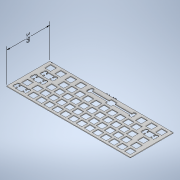
# Autodesk Inventor part: plate
Saved by Autodesk Inventor 2022 (Build 260153000, 153)
## iProperties
Created: 2022-03-03
Part Number: plate
Material: Generic
Document SubType Name: Modeling
Designer: Nathan Griffith
Density: 1 g/cm^3
Appearance: Machined - Aluminum
Author: Nathan Griffith
Autodesk Inventor part; units mm, degrees
ref_plane "YZ Plane" through (0, 0, 0) normal (1, 0, 0) x (0, 1, 0)
ref_plane "XZ Plane" through (0, 0, 0) normal (0, 1, 0) x (-1, 0, 0)
ref_plane "XY Plane" through (0, 0, 0) normal (0, 0, 1) x (1, 0, 0)
sketch "Sketch1" plane through (0, 0, 0) normal (0, 1, 0) x (-1, 0, 0)
  line L0 (0.0951, 101.505) -> (291.845, 101.505)
  line L1 (291.845, 101.505) -> (291.845, 0.2549)
  line L2 (291.845, 0.2549) -> (0.0951, 0.2549)
  line L3 (0.0951, 0.2549) -> (0.0951, 101.505)
  line L4 (127.062, 19.7804) -> (127.062, 15.0799)
  line L5 (127.062, 15.0799) -> (87.4377, 15.0799)
  line L6 (87.4377, 15.0799) -> (87.4377, 18.31)
  line L7 (87.4377, 18.31) -> (80.687, 18.31)
  line L8 (80.687, 18.31) -> (80.687, 15.0799)
  line L9 (80.687, 15.0799) -> (79.8629, 15.0799)
  line L10 (79.8629, 15.0799) -> (79.8629, 12.2811)
  line L11 (79.8629, 12.2811) -> (80.687, 12.2811)
  line L12 (80.687, 12.2811) -> (80.687, 6.011)
  line L13 (80.687, 6.011) -> (82.4121, 6.011)
  line L14 (82.4121, 6.011) -> (82.4121, 4.8107)
  line L15 (82.4121, 4.8107) -> (85.7127, 4.8107)
  line L16 (85.7127, 4.8107) -> (85.7127, 6.011)
  line L17 (85.7127, 6.011) -> (87.4377, 6.011)
  line L18 (87.4377, 6.011) -> (87.4377, 10.4813)
  line L19 (87.4377, 10.4813) -> (127.062, 10.4813)
  line L20 (127.062, 10.4813) -> (127.062, 5.7809)
  line L21 (127.062, 5.7809) -> (141.063, 5.7809)
  line L22 (141.063, 5.7809) -> (141.063, 10.4813)
  line L23 (141.063, 10.4813) -> (180.687, 10.4813)
  line L24 (180.687, 10.4813) -> (180.687, 6.011)
  line L25 (180.687, 6.011) -> (182.412, 6.011)
  line L26 (182.412, 6.011) -> (182.412, 4.8107)
  line L27 (182.412, 4.8107) -> (185.713, 4.8107)
  line L28 (185.713, 4.8107) -> (185.713, 6.011)
  line L29 (185.713, 6.011) -> (187.438, 6.011)
  line L30 (187.438, 6.011) -> (187.438, 12.2811)
  line L31 (187.438, 12.2811) -> (188.262, 12.2811)
  line L32 (188.262, 12.2811) -> (188.262, 15.0799)
  line L33 (188.262, 15.0799) -> (187.438, 15.0799)
  line L34 (187.438, 15.0799) -> (187.438, 18.31)
  line L35 (187.438, 18.31) -> (180.687, 18.31)
  line L36 (180.687, 18.31) -> (180.687, 15.0799)
  line L37 (180.687, 15.0799) -> (141.063, 15.0799)
  line L38 (141.063, 15.0799) -> (141.063, 19.7804)
  line L39 (141.063, 19.7804) -> (127.062, 19.7804)
  line L40 (269.937, 19.7804) -> (283.938, 19.7804)
  line L41 (283.938, 19.7804) -> (283.938, 5.7809)
  line L42 (283.938, 5.7809) -> (269.937, 5.7809)
  line L43 (269.937, 5.7809) -> (269.937, 19.7804)
  line L44 (246.126, 19.7804) -> (260.125, 19.7804)
  line L45 (260.125, 19.7804) -> (260.125, 5.7809)
  line L46 (260.125, 5.7809) -> (246.126, 5.7809)
  line L47 (246.126, 5.7809) -> (246.126, 19.7804)
  line L48 (222.312, 19.7804) -> (236.313, 19.7804)
  line L49 (236.313, 19.7804) -> (236.313, 5.7809)
  line L50 (236.313, 5.7809) -> (222.312, 5.7809)
  line L51 (222.312, 5.7809) -> (222.312, 19.7804)
  line L52 (198.501, 19.7804) -> (212.5, 19.7804)
  line L53 (212.5, 19.7804) -> (212.5, 5.7809)
  line L54 (212.5, 5.7809) -> (198.501, 5.7809)
  line L55 (198.501, 5.7809) -> (198.501, 19.7804)
  line L56 (55.626, 19.7804) -> (69.6253, 19.7804)
  line L57 (69.6253, 19.7804) -> (69.6253, 5.7809)
  line L58 (69.6253, 5.7809) -> (55.626, 5.7809)
  line L59 (55.626, 5.7809) -> (55.626, 19.7804)
  line L60 (31.812, 19.7804) -> (45.8128, 19.7804)
  line L61 (45.8128, 19.7804) -> (45.8128, 5.7809)
  line L62 (45.8128, 5.7809) -> (31.812, 5.7809)
  line L63 (31.812, 5.7809) -> (31.812, 19.7804)
  line L64 (8.0009, 19.7804) -> (22.0004, 19.7804)
  line L65 (22.0004, 19.7804) -> (22.0004, 5.7809)
  line L66 (22.0004, 5.7809) -> (8.0009, 5.7809)
  line L67 (8.0009, 5.7809) -> (8.0009, 19.7804)
  line L68 (255.65, 38.8303) -> (255.65, 34.1299)
  line L69 (255.65, 34.1299) -> (254.125, 34.1299)
  line L70 (254.125, 34.1299) -> (254.125, 37.3599)
  line L71 (254.125, 37.3599) -> (247.376, 37.3599)
  line L72 (247.376, 37.3599) -> (247.376, 34.1299)
  line L73 (247.376, 34.1299) -> (246.55, 34.1299)
  line L74 (246.55, 34.1299) -> (246.55, 31.3311)
  line L75 (246.55, 31.3311) -> (247.376, 31.3311)
  line L76 (247.376, 31.3311) -> (247.376, 25.061)
  line L77 (247.376, 25.061) -> (249.101, 25.061)
  line L78 (249.101, 25.061) -> (249.101, 23.8607)
  line L79 (249.101, 23.8607) -> (252.4, 23.8607)
  line L80 (252.4, 23.8607) -> (252.4, 25.061)
  line L81 (252.4, 25.061) -> (254.125, 25.061)
  line L82 (254.125, 25.061) -> (254.125, 29.53)
  line L83 (254.125, 29.53) -> (255.65, 29.53)
  line L84 (255.65, 29.53) -> (255.65, 24.8309)
  line L85 (255.65, 24.8309) -> (269.65, 24.8309)
  line L86 (269.65, 24.8309) -> (269.65, 29.53)
  line L87 (269.65, 29.53) -> (271.176, 29.53)
  line L88 (271.176, 29.53) -> (271.176, 25.061)
  line L89 (271.176, 25.061) -> (272.901, 25.061)
  line L90 (272.901, 25.061) -> (272.901, 23.8607)
  line L91 (272.901, 23.8607) -> (276.2, 23.8607)
  line L92 (276.2, 23.8607) -> (276.2, 25.061)
  line L93 (276.2, 25.061) -> (277.925, 25.061)
  line L94 (277.925, 25.061) -> (277.925, 31.3311)
  line L95 (277.925, 31.3311) -> (278.751, 31.3311)
  line L96 (278.751, 31.3311) -> (278.751, 34.1299)
  line L97 (278.751, 34.1299) -> (277.925, 34.1299)
  line L98 (277.925, 34.1299) -> (277.925, 37.3599)
  line L99 (277.925, 37.3599) -> (271.176, 37.3599)
  line L100 (271.176, 37.3599) -> (271.176, 34.1299)
  line L101 (271.176, 34.1299) -> (269.65, 34.1299)
  line L102 (269.65, 34.1299) -> (269.65, 38.8303)
  line L103 (269.65, 38.8303) -> (255.65, 38.8303)
  line L104 (17.5259, 38.8303) -> (17.5259, 34.1299)
  line L105 (17.5259, 34.1299) -> (16.0004, 34.1299)
  line L106 (16.0004, 34.1299) -> (16.0004, 37.3599)
  line L107 (16.0004, 37.3599) -> (9.2508, 37.3599)
  line L108 (9.2508, 37.3599) -> (9.2508, 34.1299)
  line L109 (9.2508, 34.1299) -> (8.4253, 34.1299)
  line L110 (8.4253, 34.1299) -> (8.4253, 31.3311)
  line L111 (8.4253, 31.3311) -> (9.2508, 31.3311)
  line L112 (9.2508, 31.3311) -> (9.2508, 25.061)
  line L113 (9.2508, 25.061) -> (10.9761, 25.061)
  line L114 (10.9761, 25.061) -> (10.9761, 23.8607)
  line L115 (10.9761, 23.8607) -> (14.2751, 23.8607)
  line L116 (14.2751, 23.8607) -> (14.2751, 25.061)
  line L117 (14.2751, 25.061) -> (16.0004, 25.061)
  line L118 (16.0004, 25.061) -> (16.0004, 29.53)
  line L119 (16.0004, 29.53) -> (17.5259, 29.53)
  line L120 (17.5259, 29.53) -> (17.5259, 24.8309)
  line L121 (17.5259, 24.8309) -> (31.5254, 24.8309)
  line L122 (31.5254, 24.8309) -> (31.5254, 29.53)
  line L123 (31.5254, 29.53) -> (33.0509, 29.53)
  line L124 (33.0509, 29.53) -> (33.0509, 25.061)
  line L125 (33.0509, 25.061) -> (34.7762, 25.061)
  line L126 (34.7762, 25.061) -> (34.7762, 23.8607)
  line L127 (34.7762, 23.8607) -> (38.0753, 23.8607)
  line L128 (38.0753, 23.8607) -> (38.0753, 25.061)
  line L129 (38.0753, 25.061) -> (39.8004, 25.061)
  line L130 (39.8004, 25.061) -> (39.8004, 31.3311)
  line L131 (39.8004, 31.3311) -> (40.6259, 31.3311)
  line L132 (40.6259, 31.3311) -> (40.6259, 34.1299)
  line L133 (40.6259, 34.1299) -> (39.8004, 34.1299)
  line L134 (39.8004, 34.1299) -> (39.8004, 37.3599)
  line L135 (39.8004, 37.3599) -> (33.0509, 37.3599)
  line L136 (33.0509, 37.3599) -> (33.0509, 34.1299)
  line L137 (33.0509, 34.1299) -> (31.5254, 34.1299)
  line L138 (31.5254, 34.1299) -> (31.5254, 38.8303)
  line L139 (31.5254, 38.8303) -> (17.5259, 38.8303)
  line L140 (219.932, 38.8303) -> (233.932, 38.8303)
  line L141 (233.932, 38.8303) -> (233.932, 24.8309)
  line L142 (233.932, 24.8309) -> (219.932, 24.8309)
  line L143 (219.932, 24.8309) -> (219.932, 38.8303)
  line L144 (200.882, 38.8303) -> (214.882, 38.8303)
  line L145 (214.882, 38.8303) -> (214.882, 24.8309)
  line L146 (214.882, 24.8309) -> (200.882, 24.8309)
  line L147 (200.882, 24.8309) -> (200.882, 38.8303)
  line L148 (181.832, 38.8303) -> (195.832, 38.8303)
  line L149 (195.832, 38.8303) -> (195.832, 24.8309)
  line L150 (195.832, 24.8309) -> (181.832, 24.8309)
  line L151 (181.832, 24.8309) -> (181.832, 38.8303)
  line L152 (162.782, 38.8303) -> (176.782, 38.8303)
  line L153 (176.782, 38.8303) -> (176.782, 24.8309)
  line L154 (176.782, 24.8309) -> (162.782, 24.8309)
  line L155 (162.782, 24.8309) -> (162.782, 38.8303)
  line L156 (143.732, 38.8303) -> (157.732, 38.8303)
  line L157 (157.732, 38.8303) -> (157.732, 24.8309)
  line L158 (157.732, 24.8309) -> (143.732, 24.8309)
  line L159 (143.732, 24.8309) -> (143.732, 38.8303)
  line L160 (124.681, 38.8303) -> (138.682, 38.8303)
  line L161 (138.682, 38.8303) -> (138.682, 24.8309)
  line L162 (138.682, 24.8309) -> (124.681, 24.8309)
  line L163 (124.681, 24.8309) -> (124.681, 38.8303)
  line L164 (105.632, 38.8303) -> (119.632, 38.8303)
  line L165 (119.632, 38.8303) -> (119.632, 24.8309)
  line L166 (119.632, 24.8309) -> (105.632, 24.8309)
  line L167 (105.632, 24.8309) -> (105.632, 38.8303)
  line L168 (86.5822, 38.8303) -> (100.582, 38.8303)
  line L169 (100.582, 38.8303) -> (100.582, 24.8309)
  line L170 (100.582, 24.8309) -> (86.5822, 24.8309)
  line L171 (86.5822, 24.8309) -> (86.5822, 38.8303)
  line L172 (67.5322, 38.8303) -> (81.5315, 38.8303)
  line L173 (81.5315, 38.8303) -> (81.5315, 24.8309)
  line L174 (81.5315, 24.8309) -> (67.5322, 24.8309)
  line L175 (67.5322, 24.8309) -> (67.5322, 38.8303)
  line L176 (48.4822, 38.8303) -> (62.4815, 38.8303)
  line L177 (62.4815, 38.8303) -> (62.4815, 24.8309)
  line L178 (62.4815, 24.8309) -> (48.4822, 24.8309)
  line L179 (48.4822, 24.8309) -> (48.4822, 38.8303)
  line L180 (260.412, 57.8803) -> (260.412, 53.1798)
  line L181 (260.412, 53.1798) -> (258.888, 53.1798)
  line L182 (258.888, 53.1798) -> (258.888, 56.4099)
  line L183 (258.888, 56.4099) -> (252.137, 56.4099)
  line L184 (252.137, 56.4099) -> (252.137, 53.1798)
  line L185 (252.137, 53.1798) -> (251.313, 53.1798)
  line L186 (251.313, 53.1798) -> (251.313, 50.3813)
  line L187 (251.313, 50.3813) -> (252.137, 50.3813)
  line L188 (252.137, 50.3813) -> (252.137, 44.111)
  line L189 (252.137, 44.111) -> (253.861, 44.111)
  line L190 (253.861, 44.111) -> (253.861, 42.9108)
  line L191 (253.861, 42.9108) -> (257.161, 42.9108)
  line L192 (257.161, 42.9108) -> (257.161, 44.111)
  line L193 (257.161, 44.111) -> (258.888, 44.111)
  line L194 (258.888, 44.111) -> (258.888, 48.58)
  line L195 (258.888, 48.58) -> (260.412, 48.58)
  line L196 (260.412, 48.58) -> (260.412, 43.881)
  line L197 (260.412, 43.881) -> (274.413, 43.881)
  line L198 (274.413, 43.881) -> (274.413, 48.58)
  line L199 (274.413, 48.58) -> (275.937, 48.58)
  line L200 (275.937, 48.58) -> (275.937, 44.111)
  line L201 (275.937, 44.111) -> (277.662, 44.111)
  line L202 (277.662, 44.111) -> (277.662, 42.9108)
  line L203 (277.662, 42.9108) -> (280.963, 42.9108)
  line L204 (280.963, 42.9108) -> (280.963, 44.111)
  line L205 (280.963, 44.111) -> (282.688, 44.111)
  line L206 (282.688, 44.111) -> (282.688, 50.3813)
  line L207 (282.688, 50.3813) -> (283.512, 50.3813)
  line L208 (283.512, 50.3813) -> (283.512, 53.1798)
  line L209 (283.512, 53.1798) -> (282.688, 53.1798)
  line L210 (282.688, 53.1798) -> (282.688, 56.4099)
  line L211 (282.688, 56.4099) -> (275.937, 56.4099)
  line L212 (275.937, 56.4099) -> (275.937, 53.1798)
  line L213 (275.937, 53.1798) -> (274.413, 53.1798)
  line L214 (274.413, 53.1798) -> (274.413, 57.8803)
  line L215 (274.413, 57.8803) -> (260.412, 57.8803)
  line L216 (229.457, 57.8803) -> (243.457, 57.8803)
  line L217 (243.457, 57.8803) -> (243.457, 43.881)
  line L218 (243.457, 43.881) -> (229.457, 43.881)
  line L219 (229.457, 43.881) -> (229.457, 57.8803)
  line L220 (210.407, 57.8803) -> (224.407, 57.8803)
  line L221 (224.407, 57.8803) -> (224.407, 43.881)
  line L222 (224.407, 43.881) -> (210.407, 43.881)
  line L223 (210.407, 43.881) -> (210.407, 57.8803)
  line L224 (191.357, 57.8803) -> (205.357, 57.8803)
  line L225 (205.357, 57.8803) -> (205.357, 43.881)
  line L226 (205.357, 43.881) -> (191.357, 43.881)
  line L227 (191.357, 43.881) -> (191.357, 57.8803)
  line L228 (172.307, 57.8803) -> (186.307, 57.8803)
  line L229 (186.307, 57.8803) -> (186.307, 43.881)
  line L230 (186.307, 43.881) -> (172.307, 43.881)
  line L231 (172.307, 43.881) -> (172.307, 57.8803)
  line L232 (153.257, 57.8803) -> (167.257, 57.8803)
  line L233 (167.257, 57.8803) -> (167.257, 43.881)
  line L234 (167.257, 43.881) -> (153.257, 43.881)
  line L235 (153.257, 43.881) -> (153.257, 57.8803)
  line L236 (134.207, 57.8803) -> (148.207, 57.8803)
  line L237 (148.207, 57.8803) -> (148.207, 43.881)
  line L238 (148.207, 43.881) -> (134.207, 43.881)
  line L239 (134.207, 43.881) -> (134.207, 57.8803)
  line L240 (115.157, 57.8803) -> (129.157, 57.8803)
  line L241 (129.157, 57.8803) -> (129.157, 43.881)
  line L242 (129.157, 43.881) -> (115.157, 43.881)
  line L243 (115.157, 43.881) -> (115.157, 57.8803)
  line L244 (96.1072, 57.8803) -> (110.107, 57.8803)
  line L245 (110.107, 57.8803) -> (110.107, 43.881)
  line L246 (110.107, 43.881) -> (96.1072, 43.881)
  line L247 (96.1072, 43.881) -> (96.1072, 57.8803)
  line L248 (77.0572, 57.8803) -> (91.0565, 57.8803)
  line L249 (91.0565, 57.8803) -> (91.0565, 43.881)
  line L250 (91.0565, 43.881) -> (77.0572, 43.881)
  line L251 (77.0572, 43.881) -> (77.0572, 57.8803)
  line L252 (58.0072, 57.8803) -> (72.0065, 57.8803)
  line L253 (72.0065, 57.8803) -> (72.0065, 43.881)
  line L254 (72.0065, 43.881) -> (58.0072, 43.881)
  line L255 (58.0072, 43.881) -> (58.0072, 57.8803)
  line L256 (38.9573, 57.8803) -> (52.9565, 57.8803)
  line L257 (52.9565, 57.8803) -> (52.9565, 43.881)
  line L258 (52.9565, 43.881) -> (38.9573, 43.881)
  line L259 (38.9573, 43.881) -> (38.9573, 57.8803)
  line L260 (12.762, 57.8803) -> (26.7629, 57.8803)
  line L261 (26.7629, 57.8803) -> (26.7629, 43.881)
  line L262 (26.7629, 43.881) -> (12.762, 43.881)
  line L263 (12.762, 43.881) -> (12.762, 57.8803)
  line L264 (267.557, 76.9303) -> (281.557, 76.9303)
  line L265 (281.557, 76.9303) -> (281.557, 62.931)
  line L266 (281.557, 62.931) -> (267.557, 62.931)
  line L267 (267.557, 62.931) -> (267.557, 76.9303)
  line L268 (243.745, 76.9303) -> (257.744, 76.9303)
  line L269 (257.744, 76.9303) -> (257.744, 62.931)
  line L270 (257.744, 62.931) -> (243.745, 62.931)
  line L271 (243.745, 62.931) -> (243.745, 76.9303)
  line L272 (224.695, 76.9303) -> (238.694, 76.9303)
  line L273 (238.694, 76.9303) -> (238.694, 62.931)
  line L274 (238.694, 62.931) -> (224.695, 62.931)
  line L275 (224.695, 62.931) -> (224.695, 76.9303)
  line L276 (205.645, 76.9303) -> (219.644, 76.9303)
  line L277 (219.644, 76.9303) -> (219.644, 62.931)
  line L278 (219.644, 62.931) -> (205.645, 62.931)
  line L279 (205.645, 62.931) -> (205.645, 76.9303)
  line L280 (186.595, 76.9303) -> (200.594, 76.9303)
  line L281 (200.594, 76.9303) -> (200.594, 62.931)
  line L282 (200.594, 62.931) -> (186.595, 62.931)
  line L283 (186.595, 62.931) -> (186.595, 76.9303)
  line L284 (167.545, 76.9303) -> (181.544, 76.9303)
  line L285 (181.544, 76.9303) -> (181.544, 62.931)
  line L286 (181.544, 62.931) -> (167.545, 62.931)
  line L287 (167.545, 62.931) -> (167.545, 76.9303)
  line L288 (148.495, 76.9303) -> (162.494, 76.9303)
  line L289 (162.494, 76.9303) -> (162.494, 62.931)
  line L290 (162.494, 62.931) -> (148.495, 62.931)
  line L291 (148.495, 62.931) -> (148.495, 76.9303)
  line L292 (129.445, 76.9303) -> (143.444, 76.9303)
  line L293 (143.444, 76.9303) -> (143.444, 62.931)
  line L294 (143.444, 62.931) -> (129.445, 62.931)
  line L295 (129.445, 62.931) -> (129.445, 76.9303)
  line L296 (110.395, 76.9303) -> (124.394, 76.9303)
  line L297 (124.394, 76.9303) -> (124.394, 62.931)
  line L298 (124.394, 62.931) -> (110.395, 62.931)
  line L299 (110.395, 62.931) -> (110.395, 76.9303)
  line L300 (91.3447, 76.9303) -> (105.344, 76.9303)
  line L301 (105.344, 76.9303) -> (105.344, 62.931)
  line L302 (105.344, 62.931) -> (91.3447, 62.931)
  line L303 (91.3447, 62.931) -> (91.3447, 76.9303)
  line L304 (72.2947, 76.9303) -> (86.294, 76.9303)
  line L305 (86.294, 76.9303) -> (86.294, 62.931)
  line L306 (86.294, 62.931) -> (72.2947, 62.931)
  line L307 (72.2947, 62.931) -> (72.2947, 76.9303)
  line L308 (53.2447, 76.9303) -> (67.244, 76.9303)
  line L309 (67.244, 76.9303) -> (67.244, 62.931)
  line L310 (67.244, 62.931) -> (53.2447, 62.931)
  line L311 (53.2447, 62.931) -> (53.2447, 76.9303)
  line L312 (34.1946, 76.9303) -> (48.194, 76.9303)
  line L313 (48.194, 76.9303) -> (48.194, 62.931)
  line L314 (48.194, 62.931) -> (34.1946, 62.931)
  line L315 (34.1946, 62.931) -> (34.1946, 76.9303)
  line L316 (10.3821, 76.9303) -> (24.3816, 76.9303)
  line L317 (24.3816, 76.9303) -> (24.3816, 62.931)
  line L318 (24.3816, 62.931) -> (10.3821, 62.931)
  line L319 (10.3821, 62.931) -> (10.3821, 76.9303)
  line L320 (262.795, 95.9817) -> (262.795, 91.2813)
  line L321 (262.795, 91.2813) -> (261.269, 91.2813)
  line L322 (261.269, 91.2813) -> (261.269, 94.5113)
  line L323 (261.269, 94.5113) -> (254.52, 94.5113)
  line L324 (254.52, 94.5113) -> (254.52, 91.2813)
  line L325 (254.52, 91.2813) -> (253.694, 91.2813)
  line L326 (253.694, 91.2813) -> (253.694, 88.4813)
  line L327 (253.694, 88.4813) -> (254.52, 88.4813)
  line L328 (254.52, 88.4813) -> (254.52, 82.211)
  line L329 (254.52, 82.211) -> (256.243, 82.211)
  line L330 (256.243, 82.211) -> (256.243, 81.0122)
  line L331 (256.243, 81.0122) -> (259.544, 81.0122)
  line L332 (259.544, 81.0122) -> (259.544, 82.211)
  line L333 (259.544, 82.211) -> (261.269, 82.211)
  line L334 (261.269, 82.211) -> (261.269, 86.68)
  line L335 (261.269, 86.68) -> (262.795, 86.68)
  line L336 (262.795, 86.68) -> (262.795, 81.981)
  line L337 (262.795, 81.981) -> (276.794, 81.981)
  line L338 (276.794, 81.981) -> (276.794, 86.68)
  line L339 (276.794, 86.68) -> (278.32, 86.68)
  line L340 (278.32, 86.68) -> (278.32, 82.211)
  line L341 (278.32, 82.211) -> (280.045, 82.211)
  line L342 (280.045, 82.211) -> (280.045, 81.0122)
  line L343 (280.045, 81.0122) -> (283.344, 81.0122)
  line L344 (283.344, 81.0122) -> (283.344, 82.211)
  line L345 (283.344, 82.211) -> (285.069, 82.211)
  line L346 (285.069, 82.211) -> (285.069, 88.4813)
  line L347 (285.069, 88.4813) -> (285.895, 88.4813)
  line L348 (285.895, 88.4813) -> (285.895, 91.2813)
  line L349 (285.895, 91.2813) -> (285.069, 91.2813)
  line L350 (285.069, 91.2813) -> (285.069, 94.5113)
  line L351 (285.069, 94.5113) -> (278.32, 94.5113)
  line L352 (278.32, 94.5113) -> (278.32, 91.2813)
  line L353 (278.32, 91.2813) -> (276.794, 91.2813)
  line L354 (276.794, 91.2813) -> (276.794, 95.9817)
  line L355 (276.794, 95.9817) -> (262.795, 95.9817)
  line L356 (234.22, 95.9817) -> (248.219, 95.9817)
  line L357 (248.219, 95.9817) -> (248.219, 81.981)
  line L358 (248.219, 81.981) -> (234.22, 81.981)
  line L359 (234.22, 81.981) -> (234.22, 95.9817)
  line L360 (215.17, 95.9817) -> (229.169, 95.9817)
  line L361 (229.169, 95.9817) -> (229.169, 81.981)
  line L362 (229.169, 81.981) -> (215.17, 81.981)
  line L363 (215.17, 81.981) -> (215.17, 95.9817)
  line L364 (196.12, 95.9817) -> (210.119, 95.9817)
  line L365 (210.119, 95.9817) -> (210.119, 81.981)
  line L366 (210.119, 81.981) -> (196.12, 81.981)
  line L367 (196.12, 81.981) -> (196.12, 95.9817)
  line L368 (177.07, 95.9817) -> (191.069, 95.9817)
  line L369 (191.069, 95.9817) -> (191.069, 81.981)
  line L370 (191.069, 81.981) -> (177.07, 81.981)
  line L371 (177.07, 81.981) -> (177.07, 95.9817)
  line L372 (158.02, 95.9817) -> (172.019, 95.9817)
  line L373 (172.019, 95.9817) -> (172.019, 81.981)
  line L374 (172.019, 81.981) -> (158.02, 81.981)
  line L375 (158.02, 81.981) -> (158.02, 95.9817)
  line L376 (138.97, 95.9817) -> (152.969, 95.9817)
  line L377 (152.969, 95.9817) -> (152.969, 81.981)
  line L378 (152.969, 81.981) -> (138.97, 81.981)
  line L379 (138.97, 81.981) -> (138.97, 95.9817)
  line L380 (119.918, 95.9817) -> (133.919, 95.9817)
  line L381 (133.919, 95.9817) -> (133.919, 81.981)
  line L382 (133.919, 81.981) -> (119.918, 81.981)
  line L383 (119.918, 81.981) -> (119.918, 95.9817)
  line L384 (100.868, 95.9817) -> (114.869, 95.9817)
  line L385 (114.869, 95.9817) -> (114.869, 81.981)
  line L386 (114.869, 81.981) -> (100.868, 81.981)
  line L387 (100.868, 81.981) -> (100.868, 95.9817)
  line L388 (81.8197, 95.9817) -> (95.819, 95.9817)
  line L389 (95.819, 95.9817) -> (95.819, 81.981)
  line L390 (95.819, 81.981) -> (81.8197, 81.981)
  line L391 (81.8197, 81.981) -> (81.8197, 95.9817)
  line L392 (62.7697, 95.9817) -> (76.769, 95.9817)
  line L393 (76.769, 95.9817) -> (76.769, 81.981)
  line L394 (76.769, 81.981) -> (62.7697, 81.981)
  line L395 (62.7697, 81.981) -> (62.7697, 95.9817)
  line L396 (43.7198, 95.9817) -> (57.719, 95.9817)
  line L397 (57.719, 95.9817) -> (57.719, 81.981)
  line L398 (57.719, 81.981) -> (43.7198, 81.981)
  line L399 (43.7198, 81.981) -> (43.7198, 95.9817)
  line L400 (24.6696, 95.9817) -> (38.669, 95.9817)
  line L401 (38.669, 95.9817) -> (38.669, 81.981)
  line L402 (38.669, 81.981) -> (24.6696, 81.981)
  line L403 (24.6696, 81.981) -> (24.6696, 95.9817)
  line L404 (5.6183, 95.9817) -> (19.6191, 95.9817)
  line L405 (19.6191, 95.9817) -> (19.6191, 81.981)
  line L406 (19.6191, 81.981) -> (5.6183, 81.981)
  line L407 (5.6183, 81.981) -> (5.6183, 95.9817)
  point P0 (0, 0)
  point P1 (0.0951, 0.2549)
  point P2 (291.845, 0.2549)
  point P3 (5.6183, 81.981)
  constraints: 816 end point
extrude "Extrusion1" add sketch "Sketch1" along normal blind 1.5
body "Solid1"
